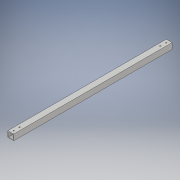
# Autodesk Inventor part: 1x1 27in
Saved by Autodesk Inventor 2018 (Build 220112000, 112)
## iProperties
Created: 2019-01-13
Part Number: 1x1 27in
Material: Generic
Document SubType Name: Modeling
Designer: s-2512711
Density: 1 g/cm^3
Appearance: Default
Author: s-2512711
Autodesk Inventor part; units mm, degrees
ref_plane "YZ Plane" through (0, 0, 0) normal (1, 0, 0) x (0, 1, 0)
ref_plane "XZ Plane" through (0, 0, 0) normal (0, 1, 0) x (-1, 0, 0)
ref_plane "XY Plane" through (0, 0, 0) normal (0, 0, 1) x (1, 0, 0)
sketch "Sketch1" plane through (0, 0, 0) normal (0, 0, 1) x (1, 0, 0)
  line L0 (0, 0) -> (25.4, 0)
  line L1 (25.4, 0) -> (25.4, 25.4)
  line L2 (25.4, 25.4) -> (0, 25.4)
  line L3 (0, 25.4) -> (0, 0)
  line L4 (3.175, 3.175) -> (22.225, 3.175)
  line L5 (22.225, 3.175) -> (22.225, 22.225)
  line L6 (22.225, 22.225) -> (3.175, 22.225)
  line L7 (3.175, 22.225) -> (3.175, 3.175)
  dimension "d0" = 25.4
  dimension "d1" = 25.4
  dimension "d2" = 3.175
  constraints: 16 end point, 4 parallel, 2 perpendicular, 1 horizontal, 3 other
  measures "d0" distance of L2.end L1.end
  measures "d1" distance of L1.end L0.end
  measures "d2" distance between parallel lines of L3 L7
extrude "Extrusion1" add sketch "Sketch1" along normal blind 685.8
sketch "Sketch2" plane through (0, 25.4, 0) normal (0, 1, 0) x (1, 0, 0)
  line L0 (25.4, 0) -> (0, 0) construction
  line L1 (12.7, 0) -> (12.7, -12.7) construction
  line L2 (12.7, -12.7) -> (12.7, -38.1) construction
  line L3 (0, 0) -> (0, -685.8) construction
  line L4 (0, -342.9) -> (25.4, -342.9) construction
  circle A0 centre (12.7, -38.1) radius 2.5797
  circle A1 centre (12.7, -12.7) radius 2.5797
  line L5 (25.4, -685.8) -> (0, -685.8) construction
  line L6 (12.7, -685.8) -> (12.7, -673.1) construction
  line L7 (12.7, -673.1) -> (12.7, -647.7) construction
  line L8 (0, -685.8) -> (0, 0) construction
  circle A2 centre (12.7, -647.7) radius 2.5797
  circle A3 centre (12.7, -673.1) radius 2.5797
  dimension "d5" = 12.7
  dimension "d6" = 25.4
  dimension "d7" = 5.1594
  constraints: 14 end point, 8 symmetric about line, 4 centre point, 4 coincident, 2 midpoint, 2 point on line, 1 horizontal, 1 vertical, 2 other
  measures "d5" distance of L1.start L1.end
  measures "d6" distance of L1.end L2.end
  measures "d7" diameter of A0
extrude "Extrusion2" cut sketch "Sketch2" against normal blind 25.4
body "Solid1"
